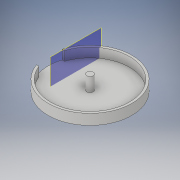
# Autodesk Inventor part: watchChargerBottom
Saved by Autodesk Inventor 2019 (Build 230136000, 136)
## iProperties
Created: 2019-12-08
Part Number: watchChargerBottom
Material: Generic
Document SubType Name: Modeling
Designer: Derek
Density: 1 g/cm^3
Appearance: Default
Author: Derek
Autodesk Inventor part; units mm, degrees
ref_plane "YZ Plane" through (0, 0, 0) normal (1, 0, 0) x (0, 1, 0)
ref_plane "XZ Plane" through (0, 0, 0) normal (0, 1, 0) x (-1, 0, 0)
ref_plane "XY Plane" through (0, 0, 0) normal (0, 0, 1) x (1, 0, 0)
sketch "Sketch1" plane through (0, 0, 0) normal (0, 1, 0) x (-1, 0, 0)
  circle A0 centre (0, 0) radius 18
  dimension "d1" = 36
  constraints: 1 centre point
  measures "d1" diameter of A0
extrude "Extrusion1" add sketch "Sketch1" along normal blind 2
sketch "Sketch2" plane through (0, 2, 0) normal (0, 1, 0) x (1, 0, 0)
  circle A0 centre (0, 0) radius 17
  dimension "d4" = 34
  constraints: 1 centre point, 1 coincident
  measures "d4" diameter of A0
extrude "Extrusion2" cut sketch "Sketch2" against normal blind 1.5
ref_plane "Work Plane1" through (-9.8347, 0.5, -3.688) normal (-1, 0, 0) x (0, 0, 1)
sketch "Sketch5" plane through (-9.8347, 0.5, -3.688) normal (-1, 0, 0) x (0, 0, 1)
  point P0 (3.688, -0.5)
ref_plane "Work Plane4" through (-9.8347, 0.5, -3.688) normal (-1, 0, 0) x (0, 0, 1)
sketch "Sketch6" plane through (-9.8347, 0.5, -3.688) normal (-1, 0, 0) x (0, 0, 1)
  line L0 (-13.312, 0) -> (20.688, 0) projected
  line L1 (21.688, 1.5) -> (-14.312, 1.5) projected
  line L2 (-1.5361, 0) -> (9.81, 0)
  line L3 (9.81, 0) -> (9.81, 1.5)
  line L4 (9.81, 1.5) -> (-1.5361, 1.5)
  line L5 (-1.5361, 1.5) -> (-1.5361, 0)
  point P0 (3.688, -0.5)
  constraints: 8 end point, 2 parallel, 2 point on line, 1 horizontal, 1 perpendicular
extrude "Extrusion4" cut sketch "Sketch6" along normal blind 15
sketch "Sketch8" plane through (0, 2, 0) normal (0, 1, 0) x (1, 0, 0)
  arc A0 (-16.9269, -6.122) -> (-17.2252, 5.2241) centre (0, 0) ccw projected
  line L0 (-15.8594, -6.122) -> (-16.9269, -6.122) projected
  line L1 (-16.9269, -6.122) -> (-15.8594, -6.122)
  arc A1 (-15.8594, -6.122) -> (-16.1774, 5.2241) centre (0, 0) ccw projected
  arc A2 (-15.8594, -6.122) -> (-16.1774, 5.2241) centre (0, 0) ccw
  arc A3 (-16.9269, -6.122) -> (-17.2252, 5.2241) centre (0, 0) ccw
  arc A4 (-17.2252, 5.2241) -> (-16.9269, -6.122) centre (0, 0) ccw projected
  line L2 (-16.1774, 5.2241) -> (-17.2252, 5.2241) projected
  line L3 (-17.2252, 5.2241) -> (-16.1774, 5.2241)
  constraints: 4 end point, 4 point on circle, 2 centre point, 2 concentric, 1 collinear, 1 horizontal
extrude "Extrusion5" add sketch "Sketch8" along normal blind 2.5 contours L0 A1 L2 A0
sketch "Sketch9" plane through (0, 0.5, 0) normal (0, 1, 0) x (1, 0, 0)
  circle A0 centre (0, 0) radius 1.3727
  constraints: 1 centre point, 1 coincident
extrude "Extrusion6" add sketch "Sketch9" along normal blind 6
body "Solid1"
